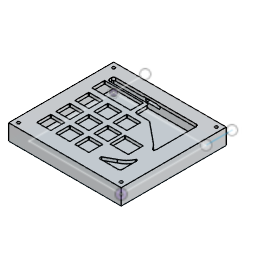
MyCroPad Case V2 (Autodesk Fusion 360 design; units mm, degrees)
part number: 2026-06-08-20-17-32-064
Autodesk Fusion 360 part; units mm, degrees
sketch "Sketch1" plane through (0, 0, 0) normal (0, 0, 1) x (1, 0, 0)
sketch "Sketch2" plane through (0, 0, 0) normal (0, 0, 1) x (1, 0, 0)
  line L0 (0, 0) -> (-92, 0)
  line L1 (-92, 0) -> (-92, 84.5)
  line L2 (-92, 84.5) -> (0, 84.5)
  line L3 (0, 84.5) -> (0, 0)
  dimension "d39" = 92
  dimension "d40" = 84.5
  constraint horizontal L0
  constraint vertical L1
  constraint horizontal L2
  constraint vertical L3
  constraint coincident L0.start L3.end
  measures "d39" distance of L0.start L0.end
  measures "d40" distance of L0.start L2.end
sketch "Sketch3" plane through (0, 0, 0) normal (0, 0, 1) x (1, 0, 0)
  line L0 (-92, 0) -> (-92, -0.4)
  line L1 (-92, 0) -> (-92.4, 0)
  line L2 (-92.4, 0) -> (-92.4, -0.4)
  line L3 (-92.4, -0.4) -> (-92, -0.4)
  line L4 (-92, -0.4) -> (0, -0.4)
  line L5 (0, -0.4) -> (0.4, -0.4)
  line L6 (0.4, -0.4) -> (0.4, 0)
  line L7 (0.4, 0) -> (0.4, 84.5)
  line L8 (0.4, 84.5) -> (0.4, 84.9)
  line L9 (0.4, 84.9) -> (0, 84.9)
  line L10 (0, 84.9) -> (-92, 84.9)
  line L11 (-92, 84.9) -> (-92.4, 84.9)
  line L12 (-92.4, 84.9) -> (-92.4, 84.5)
  line L13 (-92.4, 84.5) -> (-92.4, 0)
  dimension "d41" = 0.4
  dimension "d42" = 0.4
  dimension "d43" = 0.4
  dimension "d44" = 0.4
  dimension "d45" = 0.4
  constraint vertical L0
  constraint perpendicular L0 L1
  constraint perpendicular L1 L2
  constraint perpendicular L0 L5
  constraint perpendicular L5 L6
  constraint perpendicular L5 L7
  constraint perpendicular L5 L8
  constraint perpendicular L8 L9
  constraint perpendicular L8 L10
  constraint perpendicular L8 L11
  constraint perpendicular L10 L12
  measures "d41" distance of L0.start L0.end
  measures "d42" distance of L0.start L1.end
  measures "d43" distance of L4.end L5.end
  measures "d44" distance of L7.end L8.end
  measures "d45" distance of L10.end L11.end
sketch "Sketch4" plane through (0, 0, 0) normal (0, 0, 1) x (1, 0, 0)
  line L0 (0.4, -0.4) -> (0.4, -10.4)
  line L1 (0.4, -0.4) -> (10.4, -0.4)
  line L2 (10.4, -0.4) -> (10.4, -10.4)
  line L3 (10.4, -10.4) -> (0.4, -10.4)
  line L4 (10.4, -0.4) -> (10.4, 84.8903)
  line L5 (10.4, 84.8903) -> (10.4, 94.8903)
  line L6 (10.4, 94.8903) -> (0.4, 94.8903)
  line L7 (-92.4, 84.9) -> (-92.4, 94.9)
  line L8 (-92.4, 84.9) -> (-102.4, 84.9)
  line L9 (-92.4, -0.4) -> (-102.4, -0.4)
  line L10 (-92.4, -0.4) -> (-92.4, -10.4)
  line L11 (0.4, 94.8903) -> (-92.4, 94.9)
  line L12 (-102.4, 84.9) -> (-102.4, 94.9)
  line L13 (-102.4, 94.9) -> (-92.4, 94.9)
  line L14 (-102.4, 84.9) -> (-102.4, -0.4)
  line L15 (-102.4, -0.4) -> (-102.4, -10.4)
  line L16 (-102.4, -10.4) -> (-92.4, -10.4)
  line L17 (-92.4, -10.4) -> (0.4, -10.4)
  line L18 (-97.4, 84.9) -> (-97.4, 89.9)
  line L19 (-97.4, 89.9) -> (-92.4, 89.9)
  line L20 (-102.4, 42.25) -> (10.4, 42.2451)
  line L21 (-46, 42.2476) -> (-46, 94.8951)
  line L22 (-46, 42.2476) -> (-46, -10.4)
  circle A0 centre (-97.4, 89.9) radius 1.45
  circle A1 centre (-97.4041, -5.4004) radius 1.45
  circle A2 centre (5.4, 89.9) radius 1.45
  circle A3 centre (5.4041, -5.4004) radius 1.45
  line L23 (-92.4, -0.4) -> (-92.4, 84.9)
  line L24 (-92.4, 84.9) -> (0.4, 84.9)
  line L25 (0.4, 84.9) -> (0.4, -0.4)
  line L26 (0.4, -0.4) -> (-92.4, -0.4)
  dimension "d46" = 10
  dimension "d47" = 10
  dimension "d48" = 10
  dimension "d49" = 90
  dimension "d50" = 180
  dimension "d51" = 10
  dimension "d52" = 10
  dimension "d53" = 10
  dimension "d54" = 10
  dimension "d55" = 10
  dimension "d56" = 10
  dimension "d57" = 10
  dimension "d58" = 5
  dimension "d59" = 2.9
  constraint vertical L0
  constraint perpendicular L0 L1
  constraint perpendicular L1 L2
  constraint perpendicular L2 L6
  constraint vertical L7
  constraint perpendicular L7 L8
  constraint horizontal L9
  constraint perpendicular L9 L10
  constraint perpendicular L8 L12
  constraint perpendicular L9 L14
  constraint perpendicular L9 L15
  constraint perpendicular L0 L17
  constraint midpoint L8 L18.start
  constraint perpendicular L8 L18
  constraint midpoint L7 L19.end
  constraint midpoint L14 L20.start
  constraint midpoint L4 L20.end
  constraint midpoint L20 L21.start
  constraint midpoint L11 L21.end
  constraint midpoint L17 L22.end
  constraint coincident L18.end L19.start
  constraint symmetric L20 A0 A1
  constraint symmetric L22 A0 A2
  constraint symmetric L22 A1 A3
  constraint perpendicular L14 L24
  constraint perpendicular L1 L25
  measures "d46" distance of L0.start L0.end
  measures "d47" distance of L0.start L1.end
  measures "d48" distance of L1.end L2.end
  measures "d49" angle of L3 L4
  measures "d50" angle of L4 L5
  measures "d51" distance of L4.end L5.end
  measures "d52" distance of L5.end L6.end
  measures "d53" distance of L7.start L7.end
  measures "d54" distance of L7.start L8.end
  measures "d55" distance of L9.start L9.end
  measures "d56" distance of L9.start L10.end
  measures "d57" distance of L9.end L15.end
  measures "d58" distance of L18.start L18.end
  measures "d59" diameter of A0
extrude "Extrude1" add sketch "Sketch4" along normal blind 13 contours L0 L1 L2 L3 | L1 L4 L20 L25 | L0 L17 L22 L26 | L4 L5 L6 L11 L20 L21 L24 L25 | L10 L17 L22 L26 | L9 L10 L15 L16 | L9 L14 L20 L23 | L8 L14 L20 L23 | L7 L11 L21 L24 | L7 L8 L18 L19 A0 | L7 L8 L12 L13 L18 L19 A0
extrude "Extrude2" add sketch "Sketch3" along normal blind 3 contours L0 L1 L4 L5 L6 L7 L8 L9 L10 L11 L12 L13
ref_plane "WorkPlane1" through (-46, 42.25, 13) normal (0, 0, 1) x (1, 0, 0)
sketch "Sketch5" plane through (0, 0, 13) normal (0, 0, 1) x (1, 0, 0)
  arc A0 (-55.45, 17.5) -> (-55.95, 18) centre (-55.95, 17.5) ccw
  arc A1 (-50.4, 4.5) -> (-49.9, 4) centre (-49.9, 4.5) ccw
  arc A2 (-50.4, 23.55) -> (-49.9, 23.05) centre (-49.9, 23.55) ccw
  line L0 (-55.45, 36.55) -> (-55.45, 23.55)
  line L1 (-50.4, 17.5) -> (-50.4, 4.5)
  arc A3 (-55.95, 42.1) -> (-55.45, 42.6) centre (-55.95, 42.6) ccw
  line L2 (-74.5, 17.5) -> (-74.5, 4.5)
  line L3 (-68.95, 4) -> (-55.95, 4)
  line L4 (-68.95, 23.05) -> (-55.95, 23.05)
  line L5 (-88, 23.05) -> (-75, 23.05)
  arc A4 (-36.4, 36.55) -> (-36.9, 37.05) centre (-36.9, 36.55) ccw
  arc A5 (-49.9, 56.1) -> (-50.4, 55.6) centre (-49.9, 55.6) ccw
  line L6 (-50.4, 55.6) -> (-50.4, 42.6)
  line L7 (-33.875, 1.475) -> (-33.875, 58.625)
  line L8 (-49.9, 56.1) -> (-36.9, 56.1)
  arc A6 (-69.45, 4.5) -> (-68.95, 4) centre (-68.95, 4.5) ccw
  line L9 (-49.9, 37.05) -> (-36.9, 37.05)
  line L10 (-91.025, 1.475) -> (-33.875, 1.475)
  line L11 (-49.9, 4) -> (-36.9, 4)
  arc A7 (-36.4, 17.5) -> (-36.9, 18) centre (-36.9, 17.5) ccw
  line L12 (-49.9, 23.05) -> (-36.88, 23.05)
  arc A8 (-36.4, 55.6) -> (-36.9, 56.1) centre (-36.9, 55.6) ccw
  arc A9 (-55.95, 23.05) -> (-55.45, 23.55) centre (-55.95, 23.55) ccw
  arc A10 (-36.9, 4) -> (-36.4, 4.5) centre (-36.9, 4.5) ccw
  line L13 (-91.025, 58.625) -> (-33.875, 58.625)
  line L14 (-74.5, 55.6) -> (-74.5, 42.6)
  arc A11 (-88, 56.1) -> (-88.5, 55.6) centre (-88, 55.6) ccw
  line L15 (-68.95, 56.1) -> (-55.95, 56.1)
  arc A12 (-88.5, 42.6) -> (-88, 42.1) centre (-88, 42.6) ccw
  line L16 (-88, 37.05) -> (-75, 37.05)
  arc A13 (-75, 42.1) -> (-74.5, 42.6) centre (-75, 42.6) ccw
  line L17 (-74.5, 36.55) -> (-74.5, 23.55)
  line L18 (-69.45, 36.55) -> (-69.45, 23.55)
  arc A14 (-69.45, 42.6) -> (-68.95, 42.1) centre (-68.95, 42.6) ccw
  line L19 (-69.45, 55.6) -> (-69.45, 42.6)
  line L20 (-68.95, 37.05) -> (-55.95, 37.05)
  arc A15 (-75, 4) -> (-74.5, 4.5) centre (-75, 4.5) ccw
  arc A16 (-55.95, 4) -> (-55.45, 4.5) centre (-55.95, 4.5) ccw
  line L21 (-68.95, 18) -> (-55.95, 18)
  line L22 (-88, 4) -> (-75, 4)
  line L23 (-88, 18) -> (-75, 18)
  arc A17 (-69.45, 23.55) -> (-68.95, 23.05) centre (-68.95, 23.55) ccw
  arc A18 (-74.5, 36.55) -> (-75, 37.05) centre (-75, 36.55) ccw
  arc A19 (-36.9, 42.1) -> (-36.4, 42.6) centre (-36.9, 42.6) ccw
  line L24 (-36.4, 55.6) -> (-36.4, 42.6)
  line L25 (-88, 42.1) -> (-75, 42.1)
  line L26 (-88.5, 17.5) -> (-88.5, 4.5)
  arc A20 (-68.95, 37.05) -> (-69.45, 36.55) centre (-68.95, 36.55) ccw
  arc A21 (-88, 18) -> (-88.5, 17.5) centre (-88, 17.5) ccw
  line L27 (-49.9, 18) -> (-36.9, 18)
  line L28 (-49.9, 42.1) -> (-36.9, 42.1)
  line L29 (-36.4, 17.5) -> (-36.4, 4.5)
  line L30 (-88.5, 36.55) -> (-88.5, 23.55)
  arc A22 (-68.95, 56.1) -> (-69.45, 55.6) centre (-68.95, 55.6) ccw
  arc A23 (-74.5, 55.6) -> (-75, 56.1) centre (-75, 55.6) ccw
  arc A24 (-88, 37.05) -> (-88.5, 36.55) centre (-88, 36.55) ccw
  line L31 (-88.5, 55.6) -> (-88.5, 42.6)
  line L32 (-68.95, 42.1) -> (-55.95, 42.1)
  arc A25 (-49.9, 18) -> (-50.4, 17.5) centre (-49.9, 17.5) ccw
  arc A26 (-88.5, 4.5) -> (-88, 4) centre (-88, 4.5) ccw
  arc A27 (-55.45, 36.55) -> (-55.95, 37.05) centre (-55.95, 36.55) ccw
  line L33 (-88, 56.1) -> (-75, 56.1)
  arc A28 (-50.4, 42.6) -> (-49.9, 42.1) centre (-49.9, 42.6) ccw
  line L34 (-55.45, 17.5) -> (-55.45, 4.5)
  arc A29 (-55.45, 55.6) -> (-55.95, 56.1) centre (-55.95, 55.6) ccw
  line L35 (-91.025, 1.475) -> (-91.025, 58.625)
  arc A30 (-49.9, 37.05) -> (-50.4, 36.55) centre (-49.9, 36.55) ccw
  line L36 (-50.4, 36.55) -> (-50.4, 23.55)
  line L37 (-55.45, 55.6) -> (-55.45, 42.6)
  arc A31 (-74.5, 17.5) -> (-75, 18) centre (-75, 17.5) ccw
  line L38 (-69.45, 17.5) -> (-69.45, 4.5)
  arc A32 (-75, 23.05) -> (-74.5, 23.55) centre (-75, 23.55) ccw
  arc A33 (-68.95, 18) -> (-69.45, 17.5) centre (-68.95, 17.5) ccw
  line L39 (-36.4, 36.55) -> (-36.4, 23.4806)
  arc A34 (-36.88, 23.05) -> (-36.4, 23.4806) centre (-36.8952, 23.5498) ccw
  arc A35 (-88.5, 23.55) -> (-88, 23.05) centre (-88, 23.55) ccw
  line L40 (0, 0) -> (0, 84.5)
  line L41 (0, 84.5) -> (-92, 84.5)
  line L42 (-92, 84.5) -> (-92, 0)
  line L43 (-92, 0) -> (0, 0)
  line L44 (-92, 0) -> (-92, 1.475)
  line L45 (-92, 1.475) -> (-91.025, 1.475)
  line L46 (-91.025, 1.475) -> (-91.025, 0)
  line L47 (-32.75, 23.35) -> (-32.75, 22.35)
  line L48 (-32.75, 22.35) -> (-15.25, 22.35)
  line L49 (-15.25, 22.35) -> (-15.25, 36.55)
  line L50 (-15.25, 36.55) -> (-32.75, 36.55)
  line L51 (-32.75, 36.55) -> (-32.75, 23.35)
  line L52 (-32.75, 36.55) -> (-33.15, 36.55)
  line L53 (-32.75, 36.55) -> (-32.75, 36.95)
  line L54 (-33.15, 36.55) -> (-33.15, 22.35)
  line L55 (-32.75, 36.95) -> (-15.2499, 36.95)
  line L56 (-32.75, 36.95) -> (-32.7, 36.95)
  line L57 (-33.15, 36.5) -> (-33.15, 36.55)
  arc A36 (-32.7, 36.95) -> (-33.15, 36.5) centre (-32.7, 36.5) ccw
  line L58 (-15.25, 22.35) -> (-15.25, 21.95)
  line L59 (-15.25, 22.35) -> (-14.85, 22.35)
  line L60 (-15.3, 21.95) -> (-32.7, 21.95)
  line L61 (-33.15, 22.4) -> (-33.15, 36.55)
  line L62 (-32.75, 36.95) -> (-15.3, 36.95)
  line L63 (-14.85, 36.5) -> (-14.85, 22.4)
  arc A37 (-33.15, 22.4) -> (-32.7, 21.95) centre (-32.7, 22.4) ccw
  arc A38 (-15.3, 21.95) -> (-14.85, 22.4) centre (-15.3, 22.4) ccw
  arc A39 (-14.85, 36.5) -> (-15.3, 36.95) centre (-15.3, 36.5) ccw
  line L64 (-90.5, 61.91) -> (-52.5, 61.91)
  line L65 (-52.5, 61.91) -> (-52.5, 73.91)
  line L66 (-52.5, 73.91) -> (-90.5, 73.91)
  line L67 (-90.5, 73.91) -> (-90.5, 61.91)
  line L68 (-90.8972, 61.91) -> (-90.9, 61.91)
  line L69 (-90.5, 61.51) -> (-90.5, 61.5128)
  line L70 (-52.1028, 73.91) -> (-52.1, 73.91)
  line L71 (-52.5, 74.31) -> (-52.5, 74.3072)
  line L72 (-52.55, 74.31) -> (-90.45, 74.31)
  line L73 (-90.9, 73.86) -> (-90.9, 61.96)
  line L74 (-90.45, 61.51) -> (-52.55, 61.51)
  line L75 (-52.1, 61.96) -> (-52.1, 73.86)
  arc A40 (-90.9, 61.96) -> (-90.45, 61.51) centre (-90.45, 61.96) ccw
  arc A41 (-52.55, 61.51) -> (-52.1, 61.96) centre (-52.55, 61.96) ccw
  arc A42 (-52.1, 73.86) -> (-52.55, 74.31) centre (-52.55, 73.86) ccw
  arc A43 (-90.45, 74.31) -> (-90.9, 73.86) centre (-90.45, 73.86) ccw
  line L76 (-95, -2) -> (1.4416, -2)
  line L77 (1.4416, -2) -> (1.4416, 87.4146)
  line L78 (1.4416, 87.4146) -> (-95, 87.4146)
  line L79 (-95, 87.4146) -> (-95, -2)
  point P0 (-33.15, 36.95)
  dimension "d65" = 1.475
  dimension "d66" = 0.975
  dimension "d67" = 4.15
  dimension "d68" = 1
  dimension "d69" = 17.5
  dimension "d70" = 14.2
  dimension "d71" = 17.5
  dimension "d72" = 90
  dimension "d73" = 0.4
  dimension "d74" = 0.4
  dimension "d75" = 0.4
  dimension "d76" = 0.45
  dimension "d77" = 0.4
  dimension "d78" = 0.4
  dimension "d80" = 0.45
  dimension "d81" = 0.45
  dimension "d82" = 0.45
  dimension "d85" = 38
  dimension "d86" = 12
  dimension "d87" = 0.4
  dimension "d88" = 0.4
  dimension "d89" = 0.4
  dimension "d90" = 0.4
  dimension "d91" = 0.45
  dimension "d92" = 0.45
  dimension "d93" = 0.45
  dimension "d94" = 0.45
  constraint coincident L40.start L43.end
  constraint vertical L40
  constraint perpendicular L40 L41
  constraint perpendicular L41 L42
  constraint perpendicular L40 L43
  constraint perpendicular L43 L44
  constraint perpendicular L44 L45
  constraint coincident L43 L46.end
  constraint perpendicular L43 L46
  constraint perpendicular L47 L48
  constraint perpendicular L48 L49
  constraint perpendicular L51 L52
  constraint perpendicular L52 L53
  constraint perpendicular L52 L54
  constraint horizontal L55
  constraint perpendicular L7 L55
  constraint perpendicular L53 L56
  constraint coincident P0 L56
  constraint coincident P0 L57
  constraint tangent L56 A36
  constraint tangent L57 A36
  constraint perpendicular L48 L58
  constraint perpendicular L58 L59
  constraint horizontal L60
  constraint vertical L61
  constraint horizontal L62
  constraint vertical L63
  constraint tangent L60 A37
  constraint tangent L61 A37
  constraint tangent L63 A38
  constraint tangent L60 A38
  constraint tangent L62 A39
  constraint tangent L63 A39
  constraint horizontal L64
  constraint vertical L65
  constraint horizontal L66
  constraint vertical L67
  constraint horizontal L68
  constraint vertical L69
  constraint horizontal L70
  constraint vertical L71
  constraint horizontal L72
  constraint vertical L73
  constraint horizontal L74
  constraint vertical L75
  constraint tangent L73 A40
  constraint tangent L74 A40
  constraint tangent L74 A41
  constraint tangent L75 A41
  constraint tangent L72 A42
  constraint tangent L75 A42
  constraint tangent L73 A43
  constraint tangent L72 A43
  constraint coincident A40 L68.start
  constraint coincident A40 L69.end
  constraint coincident A42 L71.end
  constraint coincident A42 L70.start
  constraint horizontal L76
  constraint vertical L77
  constraint horizontal L78
  constraint vertical L79
  measures "d65" distance of L42.end L44.end
  measures "d66" distance of L44.end L10.start
  measures "d67" distance of A34.centre L47.start
  measures "d68" distance of L47.start L47.end
  measures "d69" distance of L47.end L48.end
  measures "d70" distance of L48.end L49.end
  measures "d71" distance of L49.end L50.end
  measures "d72" angle of L49 L50
  measures "d73" distance of L50.end L52.end
  measures "d74" distance of L50.end L53.end
  measures "d75" distance of L53.end P0
  measures "d76" radius of A36
  measures "d77" distance of L48.end L58.end
  measures "d78" distance of L48.end L59.end
  measures "d80" radius of A37
  measures "d81" radius of A38
  measures "d82" radius of A39
  measures "d85" distance of L64.start L64.end
  measures "d86" distance of L64.start L66.end
  measures "d87" distance of L64.start L68.end
  measures "d88" distance of L64.start L69.start
  measures "d89" distance of L65.end L70.end
  measures "d90" distance of L65.end L71.start
  measures "d91" radius of A40
  measures "d92" radius of A41
  measures "d93" radius of A42
  measures "d94" radius of A43
extrude "Extrude3" add sketch "Sketch5" 1 faces at (-61.4667, 91.5634, 13) along normal blind 3 contours L7 L10 L13 L35 | L40 L41 L42 L43 L45 L46 | L42 L43 L44 L45 L46 | L76 L77 L78 L79
sketch "Sketch6" plane through (0, 0, 16) normal (0, 0, 1) x (-1, 0, 0)
  circle A0 centre (97.4041, 5.4004) radius 1.45
  circle A1 centre (-5.4, -89.9) radius 1.45
  circle A2 centre (97.4, -89.9) radius 1.45
  circle A3 centre (-5.4041, 5.4004) radius 1.45
  line L0 (102.4, -94.9) -> (102.4, 10.4)
  line L1 (102.4, 10.4) -> (-10.4, 10.4)
  line L2 (-10.4, 10.4) -> (-10.4, -94.8903)
  line L3 (-10.4, -94.8903) -> (-0.4, -94.8903)
  line L4 (-0.4, -94.8903) -> (92.4, -94.9)
  line L5 (92.4, -94.9) -> (102.4, -94.9)
  arc A4 (88, -37.05) -> (88.5, -36.55) centre (88, -36.55) ccw
  line L6 (88, -37.05) -> (75, -37.05)
  arc A5 (74.5, -36.55) -> (75, -37.05) centre (75, -36.55) ccw
  line L7 (74.5, -36.55) -> (74.5, -23.55)
  arc A6 (75, -23.05) -> (74.5, -23.55) centre (75, -23.55) ccw
  line L8 (75, -23.05) -> (88, -23.05)
  arc A7 (88.5, -23.55) -> (88, -23.05) centre (88, -23.55) ccw
  line L9 (88.5, -23.55) -> (88.5, -36.55)
  arc A8 (49.9, -37.05) -> (50.4, -36.55) centre (49.9, -36.55) ccw
  line L10 (49.9, -37.05) -> (36.9, -37.05)
  arc A9 (36.4, -36.55) -> (36.9, -37.05) centre (36.9, -36.55) ccw
  line L11 (36.4, -36.55) -> (36.4, -23.4806)
  arc A10 (36.88, -23.05) -> (36.4, -23.4806) centre (36.8952, -23.5498) ccw
  line L12 (36.88, -23.05) -> (49.9, -23.05)
  arc A11 (50.4, -23.55) -> (49.9, -23.05) centre (49.9, -23.55) ccw
  line L13 (50.4, -23.55) -> (50.4, -36.55)
  arc A12 (15.3, -21.95) -> (14.85, -22.4) centre (15.3, -22.4) ccw
  line L14 (15.3, -21.95) -> (32.7, -21.95)
  arc A13 (33.15, -22.4) -> (32.7, -21.95) centre (32.7, -22.4) ccw
  line L15 (33.15, -22.4) -> (33.15, -36.55)
  line L16 (33.15, -36.55) -> (33.1472, -36.55)
  arc A14 (32.75, -36.9472) -> (33.1472, -36.55) centre (32.7, -36.5) ccw
  line L17 (32.75, -36.9472) -> (32.75, -36.95)
  line L18 (32.75, -36.95) -> (15.3, -36.95)
  arc A15 (14.85, -36.5) -> (15.3, -36.95) centre (15.3, -36.5) ccw
  line L19 (14.85, -36.5) -> (14.85, -22.4)
  arc A16 (68.95, -56.1) -> (69.45, -55.6) centre (68.95, -55.6) ccw
  line L20 (68.95, -56.1) -> (55.95, -56.1)
  arc A17 (55.45, -55.6) -> (55.95, -56.1) centre (55.95, -55.6) ccw
  line L21 (55.45, -55.6) -> (55.45, -42.6)
  arc A18 (55.95, -42.1) -> (55.45, -42.6) centre (55.95, -42.6) ccw
  line L22 (55.95, -42.1) -> (68.95, -42.1)
  arc A19 (69.45, -42.6) -> (68.95, -42.1) centre (68.95, -42.6) ccw
  line L23 (69.45, -42.6) -> (69.45, -55.6)
  line L24 (88.5, -42.6) -> (88.5, -55.6)
  arc A20 (88, -56.1) -> (88.5, -55.6) centre (88, -55.6) ccw
  line L25 (88, -56.1) -> (75, -56.1)
  arc A21 (74.5, -55.6) -> (75, -56.1) centre (75, -55.6) ccw
  line L26 (74.5, -55.6) -> (74.5, -42.6)
  arc A22 (75, -42.1) -> (74.5, -42.6) centre (75, -42.6) ccw
  line L27 (75, -42.1) -> (88, -42.1)
  arc A23 (88.5, -42.6) -> (88, -42.1) centre (88, -42.6) ccw
  arc A24 (88, -18) -> (88.5, -17.5) centre (88, -17.5) ccw
  line L28 (88, -18) -> (75, -18)
  arc A25 (74.5, -17.5) -> (75, -18) centre (75, -17.5) ccw
  line L29 (74.5, -17.5) -> (74.5, -4.5)
  arc A26 (75, -4) -> (74.5, -4.5) centre (75, -4.5) ccw
  line L30 (75, -4) -> (88, -4)
  arc A27 (88.5, -4.5) -> (88, -4) centre (88, -4.5) ccw
  line L31 (88.5, -4.5) -> (88.5, -17.5)
  arc A28 (68.95, -37.05) -> (69.45, -36.55) centre (68.95, -36.55) ccw
  line L32 (68.95, -37.05) -> (55.95, -37.05)
  arc A29 (55.45, -36.55) -> (55.95, -37.05) centre (55.95, -36.55) ccw
  line L33 (55.45, -36.55) -> (55.45, -23.55)
  arc A30 (55.95, -23.05) -> (55.45, -23.55) centre (55.95, -23.55) ccw
  line L34 (55.95, -23.05) -> (68.95, -23.05)
  arc A31 (69.45, -23.55) -> (68.95, -23.05) centre (68.95, -23.55) ccw
  line L35 (69.45, -23.55) -> (69.45, -36.55)
  arc A32 (55.45, -17.5) -> (55.95, -18) centre (55.95, -17.5) ccw
  line L36 (55.45, -17.5) -> (55.45, -4.5)
  arc A33 (55.95, -4) -> (55.45, -4.5) centre (55.95, -4.5) ccw
  line L37 (55.95, -4) -> (68.95, -4)
  arc A34 (69.45, -4.5) -> (68.95, -4) centre (68.95, -4.5) ccw
  line L38 (69.45, -4.5) -> (69.45, -17.5)
  arc A35 (68.95, -18) -> (69.45, -17.5) centre (68.95, -17.5) ccw
  line L39 (68.95, -18) -> (55.95, -18)
  arc A36 (36.4, -17.5) -> (36.9, -18) centre (36.9, -17.5) ccw
  line L40 (36.4, -17.5) -> (36.4, -4.5)
  arc A37 (36.9, -4) -> (36.4, -4.5) centre (36.9, -4.5) ccw
  line L41 (36.9, -4) -> (49.9, -4)
  arc A38 (50.4, -4.5) -> (49.9, -4) centre (49.9, -4.5) ccw
  line L42 (50.4, -4.5) -> (50.4, -17.5)
  arc A39 (49.9, -18) -> (50.4, -17.5) centre (49.9, -17.5) ccw
  line L43 (49.9, -18) -> (36.9, -18)
  arc A40 (49.9, -56.1) -> (50.4, -55.6) centre (49.9, -55.6) ccw
  line L44 (49.9, -56.1) -> (36.9, -56.1)
  arc A41 (36.4, -55.6) -> (36.9, -56.1) centre (36.9, -55.6) ccw
  line L45 (36.4, -55.6) -> (36.4, -42.6)
  arc A42 (36.9, -42.1) -> (36.4, -42.6) centre (36.9, -42.6) ccw
  line L46 (36.9, -42.1) -> (49.9, -42.1)
  arc A43 (50.4, -42.6) -> (49.9, -42.1) centre (49.9, -42.6) ccw
  line L47 (50.4, -42.6) -> (50.4, -55.6)
  arc A44 (90.45, -74.31) -> (90.9, -73.86) centre (90.45, -73.86) ccw
  line L48 (90.45, -74.31) -> (52.55, -74.31)
  arc A45 (52.1, -73.86) -> (52.55, -74.31) centre (52.55, -73.86) ccw
  line L49 (52.1, -73.86) -> (52.1, -61.96)
  arc A46 (52.55, -61.51) -> (52.1, -61.96) centre (52.55, -61.96) ccw
  line L50 (52.55, -61.51) -> (90.45, -61.51)
  arc A47 (90.9, -61.96) -> (90.45, -61.51) centre (90.45, -61.96) ccw
  line L51 (90.9, -61.96) -> (90.9, -73.86)
  line L52 (48.0423, -74) -> (48.0423, -63.51)
  line L53 (46.0423, -61.51) -> (33.8707, -61.51)
  line L54 (25.1556, -4) -> (7, -4)
  line L55 (5, -6) -> (5, -80.31)
  line L56 (7, -82.31) -> (48.0423, -82.31)
  line L57 (48.0423, -82.31) -> (89.3072, -82.31)
  line L58 (92, -84.5) -> (95.8674, -84.5) construction
  line L59 (89.3072, -82.31) -> (87.81, -82.31)
  line L60 (89.81, -80.31) -> (89.81, -78)
  line L61 (87.81, -76) -> (50.0423, -76)
  arc A48 (89.81, -78) -> (87.81, -76) centre (87.81, -78) ccw
  arc A49 (87.81, -82.31) -> (89.81, -80.31) centre (87.81, -80.31) ccw
  arc A50 (48.0423, -74) -> (50.0423, -76) centre (50.0423, -74) ccw
  arc A51 (48.0423, -63.51) -> (46.0423, -61.51) centre (46.0423, -63.51) ccw
  arc A52 (32.4565, -60.9242) -> (33.8707, -61.51) centre (33.8707, -59.51) ccw
  arc A53 (5, -80.31) -> (7, -82.31) centre (7, -80.31) ccw
  arc A54 (26.2162, -6.5607) -> (25.1556, -4) centre (25.1556, -5.5) ccw
  arc A55 (7, -4) -> (5, -6) centre (7, -6) ccw
  line L62 (32.4565, -60.9242) -> (11.5736, -43.8287)
  line L63 (26.2162, -6.5607) -> (13.5699, -13.562)
  ellipse E0 centre (24.0125, -29.45) end of major axis (5, -29.45) minor radius 19.0125 (16.0905, -12.1666) -> (12.3735, -44.4836) ccw
  spline S0 degree 5 poles (7.5537, -19.9325) (7.4837, -20.0883) (7.3454, -20.3864) (7.1429, -20.7932) (6.8828, -21.2533) (6.5754, -21.6821) (6.2874, -21.9509) (6.0205, -22.046) (5.7757, -21.9588) (5.5524, -21.6948) (5.3489, -21.2668) (5.2008, -20.8035) (5.0975, -20.3924) (5.0319, -20.0904) (5, -19.9325) knots 0 0 0 0 0 0 0.1 0.2 0.3 0.4 0.5 0.6 0.7 0.8 0.9 1 1 1 1 1 1
  spline S1 degree 5 poles (8.334, -40.2045) (8.2171, -40.0231) (7.9877, -39.6776) (7.6568, -39.2109) (7.2423, -38.6936) (6.7717, -38.2338) (6.3529, -37.9776) (5.9901, -37.9416) (5.6858, -38.1353) (5.4376, -38.5498) (5.2414, -39.1686) (5.1226, -39.8137) (5.0536, -40.3766) (5.0164, -40.7864) (5, -41) knots 0 0 0 0 0 0 0.1 0.2 0.3 0.4 0.5 0.6 0.7 0.8 0.9 1 1 1 1 1 1
  point P0 (48.0423, -61.51)
  point P1 (33.0423, -61.51)
  point P2 (6, -22)
  point P3 (6, -38)
  dimension "d97" = 15
  dimension "d103" = 2
  dimension "d105" = 1.5
  dimension "d106" = 2
  constraint perpendicular L50 L52
  constraint perpendicular L52 L53
  constraint perpendicular L40 L54
  constraint perpendicular L54 L55
  constraint perpendicular L52 L56
  constraint perpendicular L52 L57
  constraint horizontal L58
  constraint parallel L57 L59
  constraint perpendicular L59 L60
  constraint perpendicular L52 L61
  constraint tangent L60 A48
  constraint tangent L61 A48
  constraint tangent L59 A49
  constraint tangent L60 A49
  constraint equal A48 A49
  constraint tangent L61 A50
  constraint tangent L52 A50
  constraint equal A48 A50
  constraint coincident P0 L52
  constraint coincident P0 L53
  constraint tangent L52 A51
  constraint tangent L53 A51
  constraint equal A48 A51
  constraint coincident P1 L53
  constraint tangent L53 A52
  constraint equal A48 A52
  constraint tangent L55 A53
  constraint tangent L56 A53
  constraint equal A48 A53
  constraint tangent L54 A54
  constraint tangent L54 A55
  constraint tangent L55 A55
  constraint coincident L62.end E0
  constraint coincident L63.end E0
  constraint coincident E0 S0.start
  constraint coincident L55 S0.end
  constraint coincident E0 S1.start
  constraint coincident L55 S1.end
  measures "d97" distance of P0 P1
  measures "d103" radius of A48
  measures "d105" radius of A54
  measures "d106" radius of A55
extrude "Extrude4" cut sketch "Sketch6" against normal blind 3 contours L52 L53 L55 L56 L57 L60 L61 A48 A49 A50 A51 A52 A53 L62 E0 S1 | L54 L55 A54 A55 L63 E0 S0
ref_plane "WorkPlane2" through (-46, 42.25, 3) normal (0, 0, 1) x (1, 0, 0)
sketch "Sketch7" plane through (0, 0, 3) normal (0, 0, 1) x (1, 0, 0)
  line L0 (-94, -2) -> (-78, -2)
  line L1 (-78, -2) -> (-78, 13)
  line L2 (-78, 13) -> (-94, 13)
  line L3 (-94, 13) -> (-94, -2)
  constraint horizontal L0
  constraint vertical L1
  constraint horizontal L2
  constraint vertical L3
extrude "Extrude5" add sketch "Sketch7" against normal blind 3
sketch "Sketch8" plane through (0, 0, 0) normal (0, 0, -1) x (1, 0, 0)
  circle A0 centre (-97.4041, 5.4004) radius 1.45
  circle A1 centre (5.4, -89.9) radius 1.45
  circle A2 centre (-97.4, -89.9) radius 1.45
  circle A3 centre (5.4041, 5.4004) radius 1.45
  line L0 (-102.4, 10.4) -> (-102.4, -94.9)
  line L1 (-102.4, -94.9) -> (-92.4, -94.9)
  line L2 (-92.4, -94.9) -> (0.4, -94.8903)
  line L3 (0.4, -94.8903) -> (10.4, -94.8903)
  line L4 (10.4, -94.8903) -> (10.4, 10.4)
  line L5 (10.4, 10.4) -> (-102.4, 10.4)
  line L6 (0, -85) -> (0, -110.9243)
  line L7 (-92, -84.5) -> (-91.9967, -116.0077)
  point P0 (-92, -84.5)
  constraint vertical L6
  constraint coincident P0 L7.start
  constraint perpendicular L2 L7
sketch "Sketch9" plane through (0.0099, 94.8903, 0) normal (0.000105, 1, 0) x (-1, 0.000105, 0)
  line L0 (-0.3901, 0) -> (92.4099, 0)
  line L1 (92.4099, 0) -> (92.4099, 16)
  line L2 (92.4099, 16) -> (-0.3901, 16)
  line L3 (-0.3901, 16) -> (-0.3901, 0)
  line L4 (46.0765, 8.4) -> (46.025, 8.4)
  line L5 (46.625, 7.8515) -> (46.625, 7.8)
  line L6 (46.0765, 8.4) -> (46.025, 8.4)
  line L7 (46.625, 7.8) -> (46.625, 7.8515)
  line L8 (60.1735, 13) -> (60.225, 13)
  line L9 (59.625, 13.6) -> (59.625, 13.5485)
  line L10 (59.325, 13.6) -> (46.925, 13.6)
  line L11 (46.025, 12.7) -> (46.025, 8.7)
  line L12 (46.925, 7.8) -> (59.325, 7.8)
  line L13 (60.225, 8.7) -> (60.225, 12.7)
  arc A0 (46.025, 8.7) -> (46.925, 7.8) centre (46.925, 8.7) ccw
  arc A1 (46.925, 13.6) -> (46.025, 12.7) centre (46.925, 12.7) ccw
  arc A2 (59.325, 7.8) -> (60.225, 8.7) centre (59.325, 8.7) ccw
  arc A3 (60.225, 12.7) -> (59.325, 13.6) centre (59.325, 12.7) ccw
  line L14 (46.625, 7.8515) -> (46.625, 7.8)
  dimension "d130" = 0.9
  dimension "d131" = 0.9
  dimension "d132" = 0.9
  dimension "d133" = 0.9
  constraint horizontal L6
  constraint vertical L7
  constraint horizontal L8
  constraint vertical L9
  constraint horizontal L10
  constraint vertical L11
  constraint horizontal L12
  constraint vertical L13
  constraint tangent L11 A0
  constraint tangent L12 A0
  constraint tangent L11 A1
  constraint tangent L10 A1
  constraint tangent L12 A2
  constraint tangent L13 A2
  constraint tangent L10 A3
  constraint tangent L13 A3
  constraint coincident A3 L9.end
  constraint coincident A3 L8.start
  constraint coincident A0 L4.start
  constraint coincident A0 L5.start
  measures "d130" radius of A0
  measures "d131" radius of A1
  measures "d132" radius of A2
  measures "d133" radius of A3
extrude "Extrude6" cut sketch "Sketch9" against normal blind 16 contours L10 L11 L12 L13 A0 A1 A2 A3
